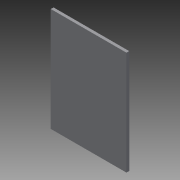
# Autodesk Inventor part: blacha pionowa ste driver
Saved by Autodesk Inventor 2015 (Build 190159000, 159)
## iProperties
Created: 2015-05-04
Part Number: blacha pionowa ste driver
Material: Ogólny
Document SubType Name: Modeling
Designer: Kuba
Density: 1 g/cm^3
Appearance: Domyślna
Author: Kuba
Autodesk Inventor part; units mm, degrees
ref_plane "YZ Plane" through (0, 0, 0) normal (1, 0, 0) x (0, 1, 0)
ref_plane "XZ Plane" through (0, 0, 0) normal (0, 1, 0) x (-1, 0, 0)
ref_plane "XY Plane" through (0, 0, 0) normal (0, 0, 1) x (1, 0, 0)
sketch "Szkic1" plane through (0, 0, 0) normal (0, 1, 0) x (-1, 0, 0)
  line L0 (-27.5, -37.75) -> (27.5, -37.75)
  line L1 (27.5, -37.75) -> (27.5, 37.75)
  line L2 (27.5, 37.75) -> (-27.5, 37.75)
  line L3 (-27.5, 37.75) -> (-27.5, -37.75)
  line L4 (-27.5, -37.75) -> (27.5, 37.75) construction
  line L5 (27.5, -37.75) -> (-27.5, 37.75) construction
  point P0 (0, 0)
  dimension "d0" = 55
  dimension "d1" = 75.5
  constraints: 12 end point, 2 midpoint, 2 parallel, 1 horizontal, 1 perpendicular
  measures "d0" distance of L2.end L1.end
  measures "d1" distance of L1.end L0.end
extrude "Wyciągnięcie proste1" add sketch "Szkic1" along normal blind 2
sketch "Szkic2" plane through (0, 0, 0) normal (0, -1, 0) x (1, 0, 0)
  line L0 (15.75, -7.5) -> (15.75, -11.75) projected
  line L1 (15.75, -11.75) -> (13, -11.75) projected
  arc A0 (13, -11.75) -> (13, -17.25) centre (13, -14.5) ccw projected
  line L2 (13, -17.25) -> (15.75, -17.25) projected
  line L3 (15.75, -17.25) -> (15.75, -21.5) projected
  line L4 (15.75, -21.5) -> (-20.25, -21.5) projected
  line L5 (-20.25, -21.5) -> (-20.25, -17.25) projected
  line L6 (-20.25, -17.25) -> (-17.5, -17.25) projected
  arc A1 (-17.5, -17.25) -> (-17.5, -11.75) centre (-17.5, -14.5) ccw projected
  line L7 (-17.5, -11.75) -> (-20.25, -11.75) projected
  line L8 (-20.25, -11.75) -> (-20.25, -7.5) projected
  line L9 (-20.25, -7.5) -> (15.75, -7.5) projected
  circle A2 centre (-17.5, -14.5) radius 1.75 projected
  circle A3 centre (19.25, -34.5) radius 1.75 projected
  circle A4 centre (-23.75, 34.5) radius 1.75 projected
  circle A5 centre (-23.75, -34.5) radius 1.75 projected
  circle A6 centre (19.25, 34.5) radius 1.75 projected
  circle A7 centre (13, -14.5) radius 1.75 projected
  line L10 (23, -37.75) -> (-27.5, -37.75) projected
  line L11 (23, 37.75) -> (23, -37.75) projected
  line L12 (-27.5, 37.75) -> (23, 37.75) projected
  line L13 (-27.5, -37.75) -> (-27.5, 37.75) projected
  line L14 (-20.25, -21.5) -> (15.75, -21.5) projected
  point P0 (0, 0)
hole "Otwór1" at (19.25, 0, 34.5) at (19.25, 0, -34.5) at (13, 0, -14.5) at (-17.5, 0, -14.5) at (-23.75, 0, -34.5) at (-23.75, 0, 34.5) direction (0, 1, 0) diameter 3.5 end through all
